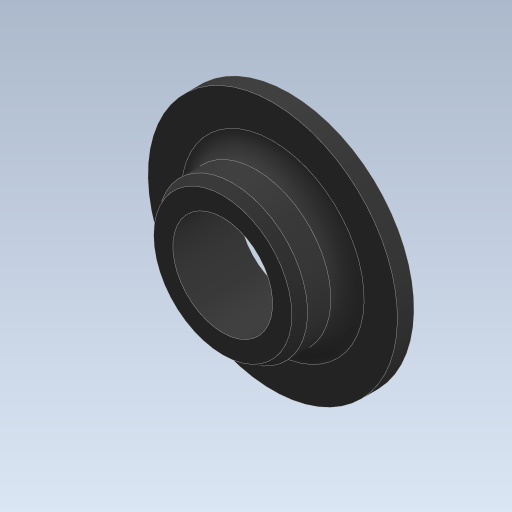
# Autodesk Inventor part: _GFM-0608-04
Saved by Autodesk Inventor 2024 (Build 280153000, 153)
## iProperties
Created: 2023-09-16
Part Number: _GFM-0608-04
Material: アセタール樹脂、黒
Document SubType Name: Modeling
Designer: michi
Density: 1.425 g/cm^3
Appearance: ゴム - 黒
Author: michi
Autodesk Inventor part; units mm, degrees
ref_plane "YZ Plane" through (0, 0, 0) normal (1, 0, 0) x (0, 1, 0)
ref_plane "XZ Plane" through (0, 0, 0) normal (0, 1, 0) x (-1, 0, 0)
ref_plane "XY Plane" through (0, 0, 0) normal (0, 0, 1) x (1, 0, 0)
sketch "スケッチ1" plane through (0, 0, 0) normal (1, 0, 0) x (0, 1, 0)
  line L0 (0, -0.4) -> (0, 2.4) construction
  line L1 (1.5, 2) -> (2.25, 2)
  line L2 (2.25, 2) -> (2.25, 0.5)
  line L3 (2.25, 0.5) -> (1.5, 0.5)
  line L4 (1.5, 0.5) -> (1.5, 2)
  line L5 (1.5, 0.5) -> (3.75, 0.5)
  line L6 (3.75, 0.5) -> (3.75, 0)
  line L7 (3.75, 0) -> (1.5, 0)
  line L8 (1.5, 0) -> (1.5, 0.5)
  point P0 (0, 0)
  point P1 (2.25, 0.5)
  dimension "d0" = 3
  dimension "d1" = 4.5
  dimension "d2" = 0.5
  dimension "d3" = 2
  dimension "d4" = 7.5
  constraints: 16 end point, 4 parallel, 2 horizontal, 2 perpendicular, 1 point on line
  measures "d0" diameter of L4 L0
  measures "d1" diameter of L2 L0
  measures "d2" distance of L5.end L6.end
  measures "d3" distance between parallel lines of L7 L1
  measures "d4" diameter of L6 L0
revolve "回転1" add sketch "スケッチ1" angle 360 about axis through (0, 0, -10) along (0, 0, 1)
fillet "フィレット1" radius 0.5 1 edges at (0, -2.25, 0.5)
chamfer "面取り1" distance 0.3 angle 30 1 edges at (0, -2.25, 2) measured on face at (0.181, 2.2427, 1.3333)
